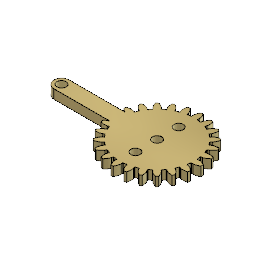
Engrenagem_v8 (Autodesk Fusion 360 design; units mm, degrees)
description: Spur Gear; Module: 1.125; Num Teeth: 24; Pressure Angle: 20.0; Backlash: 0.00 mm
Autodesk Fusion 360 part; units mm, degrees
(part 1 of 5)
sketch "Sketch1" plane through (0, 0, 0) normal (0, 1, 0) x (1, 0, 0)
sketch "Sketch1 (2)" plane through (0, 0, 0) normal (0, 0, 1) x (1, 0, 0) in component "Spur Gear (24 teeth)"
  circle A0 centre (0, 0) radius 12.0992
  circle A1 centre (0, 0) radius 1.5
extrude "Extrude1" add sketch "Sketch1 (2)" along normal blind 3 in component "Spur Gear (24 teeth)"
sketch "Sketch2" plane through (0, 0, 0) normal (0, 0, 1) x (1, 0, 0) in component "Spur Gear (24 teeth)"
  spline S0 degree 5 poles (12.6449, -1.0183) (12.6506, -1.0187) (12.6618, -1.0195) (12.6788, -1.0202) (12.7014, -1.0203) (12.7297, -1.0195) (12.758, -1.0178) (12.7864, -1.0156) (12.8147, -1.0131) (12.8431, -1.0105) (12.8715, -1.0076) (12.8999, -1.0045) (12.9284, -1.0011) (12.9568, -0.9973) (12.9852, -0.9932) (13.0137, -0.9886) (13.0421, -0.9838) (13.0705, -0.9787) (13.099, -0.9733) (13.1274, -0.9678) (13.1559, -0.962) (13.1843, -0.956) (13.2127, -0.9498) (13.2412, -0.9433) (13.2696, -0.9366) (13.298, -0.9297) (13.3264, -0.9226) (13.3549, -0.9152) (13.3833, -0.9076) (13.4117, -0.8999) (13.4401, -0.8919) (13.4684, -0.8838) (13.4968, -0.8754) (13.5252, -0.8669) (13.5535, -0.8581) (13.5819, -0.8492) (13.6102, -0.8401) (13.6385, -0.8308) (13.6669, -0.8214) (13.6952, -0.8117) (13.7234, -0.8019) (13.7517, -0.7919) (13.78, -0.7817) (13.8082, -0.7714) (13.8365, -0.7609) (13.8647, -0.7502) (13.8929, -0.7393) (13.9211, -0.7283) (13.9492, -0.7171) (13.9774, -0.7058) (14.0055, -0.6943) (14.0337, -0.6826) (14.0618, -0.6708) (14.0898, -0.6588) (14.1179, -0.6467) (14.146, -0.6344) (14.174, -0.6219) (14.202, -0.6093) (14.23, -0.5966) (14.2579, -0.5837) (14.2859, -0.5706) (14.3138, -0.5574) (14.3417, -0.544) (14.3696, -0.5305) (14.3975, -0.5169) (14.4253, -0.5031) (14.4531, -0.4891) (14.4809, -0.4751) (14.5087, -0.4608) (14.5364, -0.4465) (14.5641, -0.4319) (14.5863, -0.4202) (14.6029, -0.4114) (14.6139, -0.4054) (14.6195, -0.4024) knots 0 0 0 0 0 0 0.01428571 0.02857143 0.04285714 0.05714286 0.07142857 0.08571429 0.1 0.11428571 0.12857143 0.14285714 0.15714286 0.17142857 0.18571429 0.2 0.21428571 0.22857143 0.24285714 0.25714286 0.27142857 0.28571429 0.3 0.31428571 0.32857143 0.34285714 0.35714286 0.37142857 0.38571429 0.4 0.41428571 0.42857143 0.44285714 0.45714286 0.47142857 0.48571429 0.5 0.51428571 0.52857143 0.54285714 0.55714286 0.57142857 0.58571429 0.6 0.61428571 0.62857143 0.64285714 0.65714286 0.67142857 0.68571429 0.7 0.71428571 0.72857143 0.74285714 0.75714286 0.77142857 0.78571429 0.8 0.81428571 0.82857143 0.84285714 0.85714286 0.87142857 0.88571429 0.9 0.91428571 0.92857143 0.94285714 0.95714286 0.97142857 0.98571429 1 1 1 1 1 1
  spline S1 degree 5 poles (12.6449, 1.0183) (12.6506, 1.0187) (12.6618, 1.0195) (12.6788, 1.0202) (12.7014, 1.0203) (12.7297, 1.0195) (12.758, 1.0178) (12.7864, 1.0156) (12.8147, 1.0131) (12.8431, 1.0105) (12.8715, 1.0076) (12.8999, 1.0045) (12.9284, 1.0011) (12.9568, 0.9973) (12.9852, 0.9932) (13.0137, 0.9886) (13.0421, 0.9838) (13.0705, 0.9787) (13.099, 0.9733) (13.1274, 0.9678) (13.1559, 0.962) (13.1843, 0.956) (13.2127, 0.9498) (13.2412, 0.9433) (13.2696, 0.9366) (13.298, 0.9297) (13.3264, 0.9226) (13.3549, 0.9152) (13.3833, 0.9076) (13.4117, 0.8999) (13.4401, 0.8919) (13.4684, 0.8838) (13.4968, 0.8754) (13.5252, 0.8669) (13.5535, 0.8581) (13.5819, 0.8492) (13.6102, 0.8401) (13.6385, 0.8308) (13.6669, 0.8214) (13.6952, 0.8117) (13.7234, 0.8019) (13.7517, 0.7919) (13.78, 0.7817) (13.8082, 0.7714) (13.8365, 0.7609) (13.8647, 0.7502) (13.8929, 0.7393) (13.9211, 0.7283) (13.9492, 0.7171) (13.9774, 0.7058) (14.0055, 0.6943) (14.0337, 0.6826) (14.0618, 0.6708) (14.0898, 0.6588) (14.1179, 0.6467) (14.146, 0.6344) (14.174, 0.6219) (14.202, 0.6093) (14.23, 0.5966) (14.2579, 0.5837) (14.2859, 0.5706) (14.3138, 0.5574) (14.3417, 0.544) (14.3696, 0.5305) (14.3975, 0.5169) (14.4253, 0.5031) (14.4531, 0.4891) (14.4809, 0.4751) (14.5087, 0.4608) (14.5364, 0.4465) (14.5641, 0.4319) (14.5863, 0.4202) (14.6029, 0.4114) (14.6139, 0.4054) (14.6195, 0.4024) knots 0 0 0 0 0 0 0.01428571 0.02857143 0.04285714 0.05714286 0.07142857 0.08571429 0.1 0.11428571 0.12857143 0.14285714 0.15714286 0.17142857 0.18571429 0.2 0.21428571 0.22857143 0.24285714 0.25714286 0.27142857 0.28571429 0.3 0.31428571 0.32857143 0.34285714 0.35714286 0.37142857 0.38571429 0.4 0.41428571 0.42857143 0.44285714 0.45714286 0.47142857 0.48571429 0.5 0.51428571 0.52857143 0.54285714 0.55714286 0.57142857 0.58571429 0.6 0.61428571 0.62857143 0.64285714 0.65714286 0.67142857 0.68571429 0.7 0.71428571 0.72857143 0.74285714 0.75714286 0.77142857 0.78571429 0.8 0.81428571 0.82857143 0.84285714 0.85714286 0.87142857 0.88571429 0.9 0.91428571 0.92857143 0.94285714 0.95714286 0.97142857 0.98571429 1 1 1 1 1 1
  arc A0 (14.6195, -0.4024) -> (14.6195, 0.4024) centre (0, 0) ccw
  line L0 (12.0502, -0.9712) -> (12.6449, -1.0183)
  line L1 (12.0502, 0.9712) -> (12.6449, 1.0183)
  line L2 (12.0502, -0.9712) -> (12.0502, 0.9712)
  point P0 (12.7841, -1.0157)
  point P1 (12.9241, -1.0016)
  point P2 (13.0647, -0.9797)
  point P3 (13.2057, -0.9513)
  point P4 (13.3469, -0.9172)
  point P5 (13.4884, -0.8779)
  point P6 (13.63, -0.8336)
  point P7 (13.7716, -0.7847)
  point P8 (13.9132, -0.7313)
  point P9 (14.0548, -0.6737)
  point P10 (14.1963, -0.6119)
  point P11 (14.3376, -0.546)
  point P12 (14.4787, -0.4761)
  point P13 (12.7841, 1.0157)
  point P14 (12.9241, 1.0016)
  point P15 (13.0647, 0.9797)
  point P16 (13.2057, 0.9513)
  point P17 (13.3469, 0.9172)
  point P18 (13.4884, 0.8779)
  point P19 (13.63, 0.8336)
  point P20 (13.7716, 0.7847)
  point P21 (13.9132, 0.7313)
  point P22 (14.0548, 0.6737)
  point P23 (14.1963, 0.6119)
  point P24 (14.3376, 0.546)
  point P25 (14.4787, 0.4761)
extrude "Extrude2" add sketch "Sketch2" along normal blind 3 in component "Spur Gear (24 teeth)"
fillet "Fillet1" radius 0.1 2 edges at (12.0601, -0.972, 1.5) (12.0601, 0.972, 1.5) in component "Spur Gear (24 teeth)"
pattern_circular "C-Pattern1" count 24 over 360 about axis through (0, 0, 0) along (0, 0, 1) of "Extrude2", "Fillet1" in component "Spur Gear (24 teeth)"
sketch "Sketch3" plane through (0, 0, 0) normal (0, 0, 1) x (1, 0, 0) in component "Spur Gear (24 teeth)"
  circle A0 centre (0, 0) radius 13.5 construction
sketch "Sketch2 (2)" plane through (0, 0, 3) normal (0, 0, 1) x (1, 0, 0)
  arc A0 (11.9182, -2.0851) -> (12.0517, -1.0706) centre (0, 0) ccw
  arc A1 (12.1592, -0.9798) -> (12.0517, -1.0706) centre (12.1513, -1.0795) ccw
  line L0 (12.1592, -0.9798) -> (12.6449, -1.0183)
  spline S0 degree 5 poles (12.6449, -1.0183) (12.6506, -1.0187) (12.6618, -1.0195) (12.6788, -1.0202) (12.7014, -1.0203) (12.7297, -1.0195) (12.758, -1.0178) (12.7864, -1.0156) (12.8147, -1.0131) (12.8431, -1.0105) (12.8715, -1.0076) (12.8999, -1.0045) (12.9284, -1.0011) (12.9568, -0.9973) (12.9852, -0.9932) (13.0137, -0.9886) (13.0421, -0.9838) (13.0705, -0.9787) (13.099, -0.9733) (13.1274, -0.9678) (13.1559, -0.962) (13.1843, -0.956) (13.2127, -0.9498) (13.2412, -0.9433) (13.2696, -0.9366) (13.298, -0.9297) (13.3264, -0.9226) (13.3549, -0.9152) (13.3833, -0.9076) (13.4117, -0.8999) (13.4401, -0.8919) (13.4684, -0.8838) (13.4968, -0.8754) (13.5252, -0.8669) (13.5535, -0.8581) (13.5819, -0.8492) (13.6102, -0.8401) (13.6385, -0.8308) (13.6669, -0.8214) (13.6952, -0.8117) (13.7234, -0.8019) (13.7517, -0.7919) (13.78, -0.7817) (13.8082, -0.7714) (13.8365, -0.7609) (13.8647, -0.7502) (13.8929, -0.7393) (13.9211, -0.7283) (13.9492, -0.7171) (13.9774, -0.7058) (14.0055, -0.6943) (14.0337, -0.6826) (14.0618, -0.6708) (14.0898, -0.6588) (14.1179, -0.6467) (14.146, -0.6344) (14.174, -0.6219) (14.202, -0.6093) (14.23, -0.5966) (14.2579, -0.5837) (14.2859, -0.5706) (14.3138, -0.5574) (14.3417, -0.544) (14.3696, -0.5305) (14.3975, -0.5169) (14.4253, -0.5031) (14.4531, -0.4891) (14.4809, -0.4751) (14.5087, -0.4608) (14.5364, -0.4465) (14.5641, -0.4319) (14.5863, -0.4202) (14.6029, -0.4114) (14.6139, -0.4054) (14.6195, -0.4024) knots 0 0 0 0 0 0 0.01428571 0.02857143 0.04285714 0.05714286 0.07142857 0.08571429 0.1 0.11428571 0.12857143 0.14285714 0.15714286 0.17142857 0.18571429 0.2 0.21428571 0.22857143 0.24285714 0.25714286 0.27142857 0.28571429 0.3 0.31428571 0.32857143 0.34285714 0.35714286 0.37142857 0.38571429 0.4 0.41428571 0.42857143 0.44285714 0.45714286 0.47142857 0.48571429 0.5 0.51428571 0.52857143 0.54285714 0.55714286 0.57142857 0.58571429 0.6 0.61428571 0.62857143 0.64285714 0.65714286 0.67142857 0.68571429 0.7 0.71428571 0.72857143 0.74285714 0.75714286 0.77142857 0.78571429 0.8 0.81428571 0.82857143 0.84285714 0.85714286 0.87142857 0.88571429 0.9 0.91428571 0.92857143 0.94285714 0.95714286 0.97142857 0.98571429 1 1 1 1 1 1
  arc A2 (14.6195, -0.4024) -> (14.6195, 0.4024) centre (0, 0) ccw
  spline S1 degree 5 poles (14.6195, 0.4024) (14.6139, 0.4054) (14.6029, 0.4114) (14.5863, 0.4202) (14.5641, 0.4319) (14.5364, 0.4465) (14.5087, 0.4608) (14.4809, 0.4751) (14.4531, 0.4891) (14.4253, 0.5031) (14.3975, 0.5169) (14.3696, 0.5305) (14.3417, 0.544) (14.3138, 0.5574) (14.2859, 0.5706) (14.2579, 0.5837) (14.23, 0.5966) (14.202, 0.6093) (14.174, 0.6219) (14.146, 0.6344) (14.1179, 0.6467) (14.0898, 0.6588) (14.0618, 0.6708) (14.0337, 0.6826) (14.0055, 0.6943) (13.9774, 0.7058) (13.9492, 0.7171) (13.9211, 0.7283) (13.8929, 0.7393) (13.8647, 0.7502) (13.8365, 0.7609) (13.8082, 0.7714) (13.78, 0.7817) (13.7517, 0.7919) (13.7234, 0.8019) (13.6952, 0.8117) (13.6669, 0.8214) (13.6385, 0.8308) (13.6102, 0.8401) (13.5819, 0.8492) (13.5535, 0.8581) (13.5252, 0.8669) (13.4968, 0.8754) (13.4684, 0.8838) (13.4401, 0.8919) (13.4117, 0.8999) (13.3833, 0.9076) (13.3549, 0.9152) (13.3264, 0.9226) (13.298, 0.9297) (13.2696, 0.9366) (13.2412, 0.9433) (13.2127, 0.9498) (13.1843, 0.956) (13.1559, 0.962) (13.1274, 0.9678) (13.099, 0.9733) (13.0705, 0.9787) (13.0421, 0.9838) (13.0137, 0.9886) (12.9852, 0.9932) (12.9568, 0.9973) (12.9284, 1.0011) (12.8999, 1.0045) (12.8715, 1.0076) (12.8431, 1.0105) (12.8147, 1.0131) (12.7864, 1.0156) (12.758, 1.0178) (12.7297, 1.0195) (12.7014, 1.0203) (12.6788, 1.0202) (12.6618, 1.0195) (12.6506, 1.0187) (12.6449, 1.0183) knots -1 -1 -1 -1 -1 -1 -0.98571429 -0.97142857 -0.95714286 -0.94285714 -0.92857143 -0.91428571 -0.9 -0.88571429 -0.87142857 -0.85714286 -0.84285714 -0.82857143 -0.81428571 -0.8 -0.78571429 -0.77142857 -0.75714286 -0.74285714 -0.72857143 -0.71428571 -0.7 -0.68571429 -0.67142857 -0.65714286 -0.64285714 -0.62857143 -0.61428571 -0.6 -0.58571429 -0.57142857 -0.55714286 -0.54285714 -0.52857143 -0.51428571 -0.5 -0.48571429 -0.47142857 -0.45714286 -0.44285714 -0.42857143 -0.41428571 -0.4 -0.38571429 -0.37142857 -0.35714286 -0.34285714 -0.32857143 -0.31428571 -0.3 -0.28571429 -0.27142857 -0.25714286 -0.24285714 -0.22857143 -0.21428571 -0.2 -0.18571429 -0.17142857 -0.15714286 -0.14285714 -0.12857143 -0.11428571 -0.1 -0.08571429 -0.07142857 -0.05714286 -0.04285714 -0.02857143 -0.01428571 0 0 0 0 0 0
  line L1 (12.6449, 1.0183) -> (12.1592, 0.9798)
  arc A3 (12.0517, 1.0706) -> (12.1592, 0.9798) centre (12.1513, 1.0795) ccw
  arc A4 (12.0517, 1.0706) -> (11.9182, 2.0851) centre (0, 0) ccw
  arc A5 (11.9985, 2.2006) -> (11.9182, 2.0851) centre (12.0167, 2.1023) ccw
  line L2 (11.9985, 2.2006) -> (12.4776, 2.2892)
  spline S2 degree 5 poles (12.4776, 2.2892) (12.4832, 2.2902) (12.4943, 2.2924) (12.5108, 2.2961) (12.5327, 2.3018) (12.5598, 2.31) (12.5867, 2.3189) (12.6135, 2.3284) (12.6403, 2.3381) (12.667, 2.348) (12.6937, 2.3581) (12.7204, 2.3684) (12.747, 2.3791) (12.7734, 2.3901) (12.7998, 2.4015) (12.8261, 2.4133) (12.8523, 2.4253) (12.8785, 2.4376) (12.9046, 2.4501) (12.9306, 2.4628) (12.9566, 2.4758) (12.9825, 2.4889) (13.0083, 2.5023) (13.0341, 2.5159) (13.0599, 2.5297) (13.0855, 2.5438) (13.1111, 2.558) (13.1367, 2.5725) (13.1621, 2.5871) (13.1876, 2.602) (13.2129, 2.617) (13.2382, 2.6322) (13.2635, 2.6476) (13.2887, 2.6632) (13.3138, 2.679) (13.3389, 2.695) (13.3639, 2.7111) (13.3889, 2.7274) (13.4138, 2.7439) (13.4386, 2.7605) (13.4634, 2.7773) (13.4881, 2.7943) (13.5128, 2.8114) (13.5374, 2.8287) (13.5619, 2.8462) (13.5864, 2.8638) (13.6108, 2.8816) (13.6352, 2.8996) (13.6595, 2.9176) (13.6838, 2.9359) (13.708, 2.9543) (13.7321, 2.9728) (13.7562, 2.9915) (13.7803, 3.0104) (13.8042, 3.0294) (13.8281, 3.0485) (13.852, 3.0678) (13.8758, 3.0872) (13.8995, 3.1068) (13.9232, 3.1265) (13.9468, 3.1463) (13.9703, 3.1663) (13.9938, 3.1864) (14.0173, 3.2067) (14.0406, 3.2271) (14.064, 3.2476) (14.0872, 3.2683) (14.1104, 3.2891) (14.1336, 3.31) (14.1566, 3.3311) (14.1796, 3.3522) (14.198, 3.3693) (14.2118, 3.3822) (14.2209, 3.3908) (14.2255, 3.3951) knots 0 0 0 0 0 0 0.01428571 0.02857143 0.04285714 0.05714286 0.07142857 0.08571429 0.1 0.11428571 0.12857143 0.14285714 0.15714286 0.17142857 0.18571429 0.2 0.21428571 0.22857143 0.24285714 0.25714286 0.27142857 0.28571429 0.3 0.31428571 0.32857143 0.34285714 0.35714286 0.37142857 0.38571429 0.4 0.41428571 0.42857143 0.44285714 0.45714286 0.47142857 0.48571429 0.5 0.51428571 0.52857143 0.54285714 0.55714286 0.57142857 0.58571429 0.6 0.61428571 0.62857143 0.64285714 0.65714286 0.67142857 0.68571429 0.7 0.71428571 0.72857143 0.74285714 0.75714286 0.77142857 0.78571429 0.8 0.81428571 0.82857143 0.84285714 0.85714286 0.87142857 0.88571429 0.9 0.91428571 0.92857143 0.94285714 0.95714286 0.97142857 0.98571429 1 1 1 1 1 1
  arc A6 (14.2255, 3.3951) -> (14.0172, 4.1725) centre (0, 0) ccw
  spline S3 degree 5 poles (14.0172, 4.1725) (14.011, 4.174) (13.9988, 4.1768) (13.9805, 4.1811) (13.9561, 4.1867) (13.9255, 4.1935) (13.895, 4.2002) (13.8645, 4.2068) (13.834, 4.2132) (13.8036, 4.2195) (13.7731, 4.2256) (13.7427, 4.2316) (13.7122, 4.2374) (13.6818, 4.2431) (13.6514, 4.2486) (13.6211, 4.254) (13.5907, 4.2592) (13.5604, 4.2643) (13.53, 4.2692) (13.4998, 4.274) (13.4695, 4.2786) (13.4392, 4.2831) (13.409, 4.2874) (13.3788, 4.2915) (13.3486, 4.2955) (13.3185, 4.2993) (13.2883, 4.303) (13.2582, 4.3065) (13.2281, 4.3099) (13.1981, 4.3131) (13.1681, 4.3161) (13.1381, 4.3189) (13.1081, 4.3216) (13.0782, 4.3241) (13.0483, 4.3264) (13.0184, 4.3286) (12.9886, 4.3306) (12.9588, 4.3324) (12.929, 4.3341) (12.8993, 4.3355) (12.8696, 4.3368) (12.84, 4.3379) (12.8103, 4.3388) (12.7808, 4.3395) (12.7512, 4.3401) (12.7218, 4.3404) (12.6923, 4.3405) (12.6629, 4.3405) (12.6336, 4.3403) (12.6043, 4.3398) (12.575, 4.3391) (12.5458, 4.3383) (12.5167, 4.3371) (12.4876, 4.3358) (12.4586, 4.3342) (12.4296, 4.3324) (12.4007, 4.3304) (12.3719, 4.3282) (12.3431, 4.3258) (12.3144, 4.3231) (12.2857, 4.3201) (12.2572, 4.3168) (12.2287, 4.3131) (12.2004, 4.3091) (12.1722, 4.3047) (12.144, 4.3001) (12.1159, 4.2953) (12.0878, 4.2903) (12.0599, 4.2851) (12.0321, 4.2794) (12.0045, 4.2729) (11.9827, 4.2669) (11.9665, 4.2619) (11.9558, 4.2582) (11.9505, 4.2563) knots -1 -1 -1 -1 -1 -1 -0.98571429 -0.97142857 -0.95714286 -0.94285714 -0.92857143 -0.91428571 -0.9 -0.88571429 -0.87142857 -0.85714286 -0.84285714 -0.82857143 -0.81428571 -0.8 -0.78571429 -0.77142857 -0.75714286 -0.74285714 -0.72857143 -0.71428571 -0.7 -0.68571429 -0.67142857 -0.65714286 -0.64285714 -0.62857143 -0.61428571 -0.6 -0.58571429 -0.57142857 -0.55714286 -0.54285714 -0.52857143 -0.51428571 -0.5 -0.48571429 -0.47142857 -0.45714286 -0.44285714 -0.42857143 -0.41428571 -0.4 -0.38571429 -0.37142857 -0.35714286 -0.34285714 -0.32857143 -0.31428571 -0.3 -0.28571429 -0.27142857 -0.25714286 -0.24285714 -0.22857143 -0.21428571 -0.2 -0.18571429 -0.17142857 -0.15714286 -0.14285714 -0.12857143 -0.11428571 -0.1 -0.08571429 -0.07142857 -0.05714286 -0.04285714 -0.02857143 -0.01428571 0 0 0 0 0 0
  line L3 (11.9505, 4.2563) -> (11.4913, 4.0935)
  arc A7 (11.364, 4.1534) -> (11.4913, 4.0935) centre (11.4579, 4.1877) ccw
  arc A8 (11.364, 4.1534) -> (10.9724, 5.0987) centre (0, 0) ccw
  arc A9 (11.0201, 5.2311) -> (10.9724, 5.0987) centre (11.0631, 5.1408) ccw
  line L4 (11.0201, 5.2311) -> (11.46, 5.4406)
  spline S4 degree 5 poles (11.46, 5.4406) (11.4651, 5.443) (11.4752, 5.448) (11.4902, 5.4559) (11.5099, 5.4671) (11.534, 5.482) (11.5577, 5.4976) (11.5811, 5.5137) (11.6045, 5.53) (11.6277, 5.5465) (11.6509, 5.5631) (11.674, 5.58) (11.6969, 5.5972) (11.7196, 5.6147) (11.7421, 5.6325) (11.7645, 5.6507) (11.7867, 5.6691) (11.8087, 5.6877) (11.8307, 5.7066) (11.8526, 5.7256) (11.8743, 5.7448) (11.8959, 5.7642) (11.9175, 5.7838) (11.9389, 5.8036) (11.9601, 5.8236) (11.9813, 5.8439) (12.0023, 5.8643) (12.0232, 5.8848) (12.0441, 5.9056) (12.0648, 5.9265) (12.0854, 5.9476) (12.1059, 5.9689) (12.1263, 5.9903) (12.1466, 6.0119) (12.1668, 6.0336) (12.1869, 6.0555) (12.2069, 6.0775) (12.2267, 6.0998) (12.2465, 6.1221) (12.2662, 6.1446) (12.2858, 6.1673) (12.3053, 6.1901) (12.3247, 6.213) (12.344, 6.2361) (12.3632, 6.2593) (12.3822, 6.2827) (12.4012, 6.3062) (12.4202, 6.3298) (12.439, 6.3536) (12.4577, 6.3775) (12.4763, 6.4015) (12.4948, 6.4257) (12.5132, 6.45) (12.5316, 6.4744) (12.5498, 6.4989) (12.5679, 6.5236) (12.586, 6.5484) (12.6039, 6.5733) (12.6218, 6.5983) (12.6396, 6.6235) (12.6572, 6.6488) (12.6748, 6.6742) (12.6923, 6.6997) (12.7097, 6.7253) (12.727, 6.7511) (12.7442, 6.777) (12.7613, 6.8029) (12.7783, 6.829) (12.7953, 6.8552) (12.8121, 6.8816) (12.8289, 6.908) (12.8422, 6.9292) (12.8521, 6.9452) (12.8587, 6.9559) (12.862, 6.9612) knots 0 0 0 0 0 0 0.01428571 0.02857143 0.04285714 0.05714286 0.07142857 0.08571429 0.1 0.11428571 0.12857143 0.14285714 0.15714286 0.17142857 0.18571429 0.2 0.21428571 0.22857143 0.24285714 0.25714286 0.27142857 0.28571429 0.3 0.31428571 0.32857143 0.34285714 0.35714286 0.37142857 0.38571429 0.4 0.41428571 0.42857143 0.44285714 0.45714286 0.47142857 0.48571429 0.5 0.51428571 0.52857143 0.54285714 0.55714286 0.57142857 0.58571429 0.6 0.61428571 0.62857143 0.64285714 0.65714286 0.67142857 0.68571429 0.7 0.71428571 0.72857143 0.74285714 0.75714286 0.77142857 0.78571429 0.8 0.81428571 0.82857143 0.84285714 0.85714286 0.87142857 0.88571429 0.9 0.91428571 0.92857143 0.94285714 0.95714286 0.97142857 0.98571429 1 1 1 1 1 1
  arc A10 (12.862, 6.9612) -> (12.4596, 7.6583) centre (0, 0) ccw
  spline S5 degree 5 poles (12.4596, 7.6583) (12.4533, 7.6581) (12.4408, 7.6577) (12.422, 7.657) (12.3969, 7.6561) (12.3657, 7.6548) (12.3344, 7.6534) (12.3033, 7.6519) (12.2722, 7.6502) (12.2411, 7.6483) (12.2101, 7.6464) (12.1792, 7.6442) (12.1483, 7.642) (12.1174, 7.6396) (12.0866, 7.6371) (12.0559, 7.6344) (12.0252, 7.6316) (11.9946, 7.6287) (11.9641, 7.6256) (11.9336, 7.6224) (11.9031, 7.619) (11.8728, 7.6155) (11.8424, 7.6118) (11.8122, 7.608) (11.782, 7.604) (11.7519, 7.5999) (11.7218, 7.5957) (11.6918, 7.5913) (11.6619, 7.5867) (11.6321, 7.582) (11.6023, 7.5771) (11.5726, 7.5721) (11.543, 7.567) (11.5134, 7.5617) (11.4839, 7.5562) (11.4545, 7.5505) (11.4252, 7.5447) (11.3959, 7.5388) (11.3667, 7.5327) (11.3376, 7.5264) (11.3086, 7.5199) (11.2797, 7.5133) (11.2509, 7.5065) (11.2221, 7.4996) (11.1935, 7.4924) (11.1649, 7.4851) (11.1364, 7.4777) (11.108, 7.47) (11.0798, 7.4622) (11.0516, 7.4542) (11.0235, 7.4459) (10.9955, 7.4375) (10.9677, 7.4289) (10.9399, 7.4201) (10.9123, 7.411) (10.8848, 7.4018) (10.8574, 7.3924) (10.8301, 7.3828) (10.8029, 7.373) (10.7759, 7.363) (10.749, 7.3527) (10.7222, 7.3421) (10.6957, 7.3312) (10.6694, 7.3199) (10.6433, 7.3084) (10.6172, 7.2967) (10.5913, 7.2848) (10.5655, 7.2727) (10.5399, 7.2604) (10.5145, 7.2477) (10.4896, 7.2343) (10.4701, 7.2229) (10.4557, 7.2138) (10.4463, 7.2075) (10.4417, 7.2043) knots -1 -1 -1 -1 -1 -1 -0.98571429 -0.97142857 -0.95714286 -0.94285714 -0.92857143 -0.91428571 -0.9 -0.88571429 -0.87142857 -0.85714286 -0.84285714 -0.82857143 -0.81428571 -0.8 -0.78571429 -0.77142857 -0.75714286 -0.74285714 -0.72857143 -0.71428571 -0.7 -0.68571429 -0.67142857 -0.65714286 -0.64285714 -0.62857143 -0.61428571 -0.6 -0.58571429 -0.57142857 -0.55714286 -0.54285714 -0.52857143 -0.51428571 -0.5 -0.48571429 -0.47142857 -0.45714286 -0.44285714 -0.42857143 -0.41428571 -0.4 -0.38571429 -0.37142857 -0.35714286 -0.34285714 -0.32857143 -0.31428571 -0.3 -0.28571429 -0.27142857 -0.25714286 -0.24285714 -0.22857143 -0.21428571 -0.2 -0.18571429 -0.17142857 -0.15714286 -0.14285714 -0.12857143 -0.11428571 -0.1 -0.08571429 -0.07142857 -0.05714286 -0.04285714 -0.02857143 -0.01428571 0 0 0 0 0 0
  line L5 (10.4417, 7.2043) -> (10.0403, 6.9282)
  arc A11 (9.9018, 6.9531) -> (10.0403, 6.9282) centre (9.9836, 7.0105) ccw
  arc A12 (9.9018, 6.9531) -> (9.2789, 7.7648) centre (0, 0) ccw
  arc A13 (9.2907, 7.905) -> (9.2789, 7.7648) centre (9.3556, 7.829) ccw
  line L6 (9.2907, 7.905) -> (9.6613, 8.2213)
  spline S6 degree 5 poles (9.6613, 8.2213) (9.6656, 8.225) (9.6741, 8.2324) (9.6866, 8.2439) (9.7027, 8.2597) (9.7221, 8.2804) (9.741, 8.3016) (9.7595, 8.3232) (9.7778, 8.345) (9.796, 8.367) (9.8141, 8.3891) (9.832, 8.4113) (9.8496, 8.4338) (9.8671, 8.4566) (9.8842, 8.4797) (9.9011, 8.503) (9.9178, 8.5265) (9.9343, 8.5503) (9.9506, 8.5741) (9.9668, 8.5982) (9.9828, 8.6224) (9.9987, 8.6467) (10.0144, 8.6712) (10.03, 8.6959) (10.0453, 8.7207) (10.0605, 8.7457) (10.0756, 8.7709) (10.0904, 8.7962) (10.1052, 8.8216) (10.1198, 8.8472) (10.1342, 8.8729) (10.1485, 8.8987) (10.1627, 8.9247) (10.1767, 8.9508) (10.1906, 8.977) (10.2043, 9.0033) (10.2179, 9.0298) (10.2314, 9.0564) (10.2447, 9.0831) (10.2579, 9.11) (10.271, 9.1369) (10.2839, 9.164) (10.2967, 9.1912) (10.3093, 9.2185) (10.3219, 9.2459) (10.3343, 9.2734) (10.3465, 9.301) (10.3587, 9.3287) (10.3707, 9.3565) (10.3826, 9.3845) (10.3943, 9.4125) (10.406, 9.4406) (10.4175, 9.4688) (10.4289, 9.4972) (10.4401, 9.5256) (10.4513, 9.5541) (10.4623, 9.5828) (10.4732, 9.6115) (10.4839, 9.6403) (10.4946, 9.6692) (10.5051, 9.6982) (10.5155, 9.7273) (10.5258, 9.7564) (10.536, 9.7857) (10.546, 9.815) (10.556, 9.8445) (10.5658, 9.874) (10.5754, 9.9036) (10.585, 9.9333) (10.5945, 9.9631) (10.6038, 9.993) (10.6112, 10.0169) (10.6167, 10.0349) (10.6203, 10.0469) (10.6221, 10.0529) knots 0 0 0 0 0 0 0.01428571 0.02857143 0.04285714 0.05714286 0.07142857 0.08571429 0.1 0.11428571 0.12857143 0.14285714 0.15714286 0.17142857 0.18571429 0.2 0.21428571 0.22857143 0.24285714 0.25714286 0.27142857 0.28571429 0.3 0.31428571 0.32857143 0.34285714 0.35714286 0.37142857 0.38571429 0.4 0.41428571 0.42857143 0.44285714 0.45714286 0.47142857 0.48571429 0.5 0.51428571 0.52857143 0.54285714 0.55714286 0.57142857 0.58571429 0.6 0.61428571 0.62857143 0.64285714 0.65714286 0.67142857 0.68571429 0.7 0.71428571 0.72857143 0.74285714 0.75714286 0.77142857 0.78571429 0.8 0.81428571 0.82857143 0.84285714 0.85714286 0.87142857 0.88571429 0.9 0.91428571 0.92857143 0.94285714 0.95714286 0.97142857 0.98571429 1 1 1 1 1 1
  arc A14 (10.6221, 10.0529) -> (10.0529, 10.6221) centre (0, 0) ccw
  spline S7 degree 5 poles (10.0529, 10.6221) (10.0469, 10.6203) (10.0349, 10.6167) (10.0169, 10.6112) (9.993, 10.6038) (9.9631, 10.5945) (9.9333, 10.585) (9.9036, 10.5754) (9.874, 10.5658) (9.8445, 10.556) (9.815, 10.546) (9.7857, 10.536) (9.7564, 10.5258) (9.7273, 10.5155) (9.6982, 10.5051) (9.6692, 10.4946) (9.6403, 10.4839) (9.6115, 10.4732) (9.5828, 10.4623) (9.5541, 10.4513) (9.5256, 10.4401) (9.4972, 10.4289) (9.4688, 10.4175) (9.4406, 10.406) (9.4125, 10.3943) (9.3845, 10.3826) (9.3565, 10.3707) (9.3287, 10.3587) (9.301, 10.3465) (9.2734, 10.3343) (9.2459, 10.3219) (9.2185, 10.3093) (9.1912, 10.2967) (9.164, 10.2839) (9.1369, 10.271) (9.11, 10.2579) (9.0831, 10.2447) (9.0564, 10.2314) (9.0298, 10.2179) (9.0033, 10.2043) (8.977, 10.1906) (8.9508, 10.1767) (8.9247, 10.1627) (8.8987, 10.1485) (8.8729, 10.1342) (8.8472, 10.1198) (8.8216, 10.1052) (8.7962, 10.0904) (8.7709, 10.0756) (8.7457, 10.0605) (8.7207, 10.0453) (8.6959, 10.03) (8.6712, 10.0144) (8.6467, 9.9987) (8.6224, 9.9828) (8.5982, 9.9668) (8.5741, 9.9506) (8.5503, 9.9343) (8.5265, 9.9178) (8.503, 9.9011) (8.4797, 9.8842) (8.4566, 9.8671) (8.4338, 9.8496) (8.4113, 9.832) (8.3891, 9.8141) (8.367, 9.796) (8.345, 9.7778) (8.3232, 9.7595) (8.3016, 9.741) (8.2804, 9.7221) (8.2597, 9.7027) (8.2439, 9.6866) (8.2324, 9.6741) (8.225, 9.6656) (8.2213, 9.6613) knots -1 -1 -1 -1 -1 -1 -0.98571429 -0.97142857 -0.95714286 -0.94285714 -0.92857143 -0.91428571 -0.9 -0.88571429 -0.87142857 -0.85714286 -0.84285714 -0.82857143 -0.81428571 -0.8 -0.78571429 -0.77142857 -0.75714286 -0.74285714 -0.72857143 -0.71428571 -0.7 -0.68571429 -0.67142857 -0.65714286 -0.64285714 -0.62857143 -0.61428571 -0.6 -0.58571429 -0.57142857 -0.55714286 -0.54285714 -0.52857143 -0.51428571 -0.5 -0.48571429 -0.47142857 -0.45714286 -0.44285714 -0.42857143 -0.41428571 -0.4 -0.38571429 -0.37142857 -0.35714286 -0.34285714 -0.32857143 -0.31428571 -0.3 -0.28571429 -0.27142857 -0.25714286 -0.24285714 -0.22857143 -0.21428571 -0.2 -0.18571429 -0.17142857 -0.15714286 -0.14285714 -0.12857143 -0.11428571 -0.1 -0.08571429 -0.07142857 -0.05714286 -0.04285714 -0.02857143 -0.01428571 0 0 0 0 0 0
  line L7 (8.2213, 9.6613) -> (7.905, 9.2907)
  arc A15 (7.7648, 9.2789) -> (7.905, 9.2907) centre (7.829, 9.3556) ccw
  arc A16 (7.7648, 9.2789) -> (6.9531, 9.9018) centre (0, 0) ccw
  arc A17 (6.9282, 10.0403) -> (6.9531, 9.9018) centre (7.0105, 9.9836) ccw
  line L8 (6.9282, 10.0403) -> (7.2043, 10.4417)
  spline S8 degree 5 poles (7.2043, 10.4417) (7.2075, 10.4463) (7.2138, 10.4557) (7.2229, 10.4701) (7.2343, 10.4896) (7.2477, 10.5145) (7.2604, 10.5399) (7.2727, 10.5655) (7.2848, 10.5913) (7.2967, 10.6172) (7.3084, 10.6433) (7.3199, 10.6694) (7.3312, 10.6957) (7.3421, 10.7222) (7.3527, 10.749) (7.363, 10.7759) (7.373, 10.8029) (7.3828, 10.8301) (7.3924, 10.8574) (7.4018, 10.8848) (7.411, 10.9123) (7.4201, 10.9399) (7.4289, 10.9677) (7.4375, 10.9955) (7.4459, 11.0235) (7.4542, 11.0516) (7.4622, 11.0798) (7.47, 11.108) (7.4777, 11.1364) (7.4851, 11.1649) (7.4924, 11.1935) (7.4996, 11.2221) (7.5065, 11.2509) (7.5133, 11.2797) (7.5199, 11.3086) (7.5264, 11.3376) (7.5327, 11.3667) (7.5388, 11.3959) (7.5447, 11.4252) (7.5505, 11.4545) (7.5562, 11.4839) (7.5617, 11.5134) (7.567, 11.543) (7.5721, 11.5726) (7.5771, 11.6023) (7.582, 11.6321) (7.5867, 11.6619) (7.5913, 11.6918) (7.5957, 11.7218) (7.5999, 11.7519) (7.604, 11.782) (7.608, 11.8122) (7.6118, 11.8424) (7.6155, 11.8728) (7.619, 11.9031) (7.6224, 11.9336) (7.6256, 11.9641) (7.6287, 11.9946) (7.6316, 12.0252) (7.6344, 12.0559) (7.6371, 12.0866) (7.6396, 12.1174) (7.642, 12.1483) (7.6442, 12.1792) (7.6464, 12.2101) (7.6483, 12.2411) (7.6502, 12.2722) (7.6519, 12.3033) (7.6534, 12.3344) (7.6548, 12.3657) (7.6561, 12.3969) (7.657, 12.422) (7.6577, 12.4408) (7.6581, 12.4533) (7.6583, 12.4596) knots 0 0 0 0 0 0 0.01428571 0.02857143 0.04285714 0.05714286 0.07142857 0.08571429 0.1 0.11428571 0.12857143 0.14285714 0.15714286 0.17142857 0.18571429 0.2 0.21428571 0.22857143 0.24285714 0.25714286 0.27142857 0.28571429 0.3 0.31428571 0.32857143 0.34285714 0.35714286 0.37142857 0.38571429 0.4 0.41428571 0.42857143 0.44285714 0.45714286 0.47142857 0.48571429 0.5 0.51428571 0.52857143 0.54285714 0.55714286 0.57142857 0.58571429 0.6 0.61428571 0.62857143 0.64285714 0.65714286 0.67142857 0.68571429 0.7 0.71428571 0.72857143 0.74285714 0.75714286 0.77142857 0.78571429 0.8 0.81428571 0.82857143 0.84285714 0.85714286 0.87142857 0.88571429 0.9 0.91428571 0.92857143 0.94285714 0.95714286 0.97142857 0.98571429 1 1 1 1 1 1
  arc A18 (7.6583, 12.4596) -> (6.9612, 12.862) centre (0, 0) ccw
  spline S9 degree 5 poles (6.9612, 12.862) (6.9559, 12.8587) (6.9452, 12.8521) (6.9292, 12.8422) (6.908, 12.8289) (6.8816, 12.8121) (6.8552, 12.7953) (6.829, 12.7783) (6.8029, 12.7613) (6.777, 12.7442) (6.7511, 12.727) (6.7253, 12.7097) (6.6997, 12.6923) (6.6742, 12.6748) (6.6488, 12.6572) (6.6235, 12.6396) (6.5983, 12.6218) (6.5733, 12.6039) (6.5484, 12.586) (6.5236, 12.5679) (6.4989, 12.5498) (6.4744, 12.5316) (6.45, 12.5132) (6.4257, 12.4948) (6.4015, 12.4763) (6.3775, 12.4577) (6.3536, 12.439) (6.3298, 12.4202) (6.3062, 12.4012) (6.2827, 12.3822) (6.2593, 12.3632) (6.2361, 12.344) (6.213, 12.3247) (6.1901, 12.3053) (6.1673, 12.2858) (6.1446, 12.2662) (6.1221, 12.2465) (6.0998, 12.2267) (6.0775, 12.2069) (6.0555, 12.1869) (6.0336, 12.1668) (6.0119, 12.1466) (5.9903, 12.1263) (5.9689, 12.1059) (5.9476, 12.0854) (5.9265, 12.0648) (5.9056, 12.0441) (5.8848, 12.0232) (5.8643, 12.0023) (5.8439, 11.9813) (5.8236, 11.9601) (5.8036, 11.9389) (5.7838, 11.9175) (5.7642, 11.8959) (5.7448, 11.8743) (5.7256, 11.8526) (5.7066, 11.8307) (5.6877, 11.8087) (5.6691, 11.7867) (5.6507, 11.7645) (5.6325, 11.7421) (5.6147, 11.7196) (5.5972, 11.6969) (5.58, 11.674) (5.5631, 11.6509) (5.5465, 11.6277) (5.53, 11.6045) (5.5137, 11.5811) (5.4976, 11.5577) (5.482, 11.534) (5.4671, 11.5099) (5.4559, 11.4902) (5.448, 11.4752) (5.443, 11.4651) (5.4406, 11.46) knots -1 -1 -1 -1 -1 -1 -0.98571429 -0.97142857 -0.95714286 -0.94285714 -0.92857143 -0.91428571 -0.9 -0.88571429 -0.87142857 -0.85714286 -0.84285714 -0.82857143 -0.81428571 -0.8 -0.78571429 -0.77142857 -0.75714286 -0.74285714 -0.72857143 -0.71428571 -0.7 -0.68571429 -0.67142857 -0.65714286 -0.64285714 -0.62857143 -0.61428571 -0.6 -0.58571429 -0.57142857 -0.55714286 -0.54285714 -0.52857143 -0.51428571 -0.5 -0.48571429 -0.47142857 -0.45714286 -0.44285714 -0.42857143 -0.41428571 -0.4 -0.38571429 -0.37142857 -0.35714286 -0.34285714 -0.32857143 -0.31428571 -0.3 -0.28571429 -0.27142857 -0.25714286 -0.24285714 -0.22857143 -0.21428571 -0.2 -0.18571429 -0.17142857 -0.15714286 -0.14285714 -0.12857143 -0.11428571 -0.1 -0.08571429 -0.07142857 -0.05714286 -0.04285714 -0.02857143 -0.01428571 0 0 0 0 0 0
  line L9 (5.4406, 11.46) -> (5.2311, 11.0201)
  arc A19 (5.0987, 10.9724) -> (5.2311, 11.0201) centre (5.1408, 11.0631) ccw
  arc A20 (5.0987, 10.9724) -> (4.1534, 11.364) centre (0, 0) ccw
  arc A21 (4.0935, 11.4913) -> (4.1534, 11.364) centre (4.1877, 11.4579) ccw
  line L10 (4.0935, 11.4913) -> (4.2563, 11.9505)
  spline S10 degree 5 poles (4.2563, 11.9505) (4.2582, 11.9558) (4.2619, 11.9665) (4.2669, 11.9827) (4.2729, 12.0045) (4.2794, 12.0321) (4.2851, 12.0599) (4.2903, 12.0878) (4.2953, 12.1159) (4.3001, 12.144) (4.3047, 12.1722) (4.3091, 12.2004) (4.3131, 12.2287) (4.3168, 12.2572) (4.3201, 12.2857) (4.3231, 12.3144) (4.3258, 12.3431) (4.3282, 12.3719) (4.3304, 12.4007) (4.3324, 12.4296) (4.3342, 12.4586) (4.3358, 12.4876) (4.3371, 12.5167) (4.3383, 12.5458) (4.3391, 12.575) (4.3398, 12.6043) (4.3403, 12.6336) (4.3405, 12.6629) (4.3405, 12.6923) (4.3404, 12.7218) (4.3401, 12.7512) (4.3395, 12.7808) (4.3388, 12.8103) (4.3379, 12.84) (4.3368, 12.8696) (4.3355, 12.8993) (4.3341, 12.929) (4.3324, 12.9588) (4.3306, 12.9886) (4.3286, 13.0184) (4.3264, 13.0483) (4.3241, 13.0782) (4.3216, 13.1081) (4.3189, 13.1381) (4.3161, 13.1681) (4.3131, 13.1981) (4.3099, 13.2281) (4.3065, 13.2582) (4.303, 13.2883) (4.2993, 13.3185) (4.2955, 13.3486) (4.2915, 13.3788) (4.2874, 13.409) (4.2831, 13.4392) (4.2786, 13.4695) (4.274, 13.4998) (4.2692, 13.53) (4.2643, 13.5604) (4.2592, 13.5907) (4.254, 13.6211) (4.2486, 13.6514) (4.2431, 13.6818) (4.2374, 13.7122) (4.2316, 13.7427) (4.2256, 13.7731) (4.2195, 13.8036) (4.2132, 13.834) (4.2068, 13.8645) (4.2002, 13.895) (4.1935, 13.9255) (4.1867, 13.9561) (4.1811, 13.9805) (4.1768, 13.9988) (4.174, 14.011) (4.1725, 14.0172) knots 0 0 0 0 0 0 0.01428571 0.02857143 0.04285714 0.05714286 0.07142857 0.08571429 0.1 0.11428571 0.12857143 0.14285714 0.15714286 0.17142857 0.18571429 0.2 0.21428571 0.22857143 0.24285714 0.25714286 0.27142857 0.28571429 0.3 0.31428571 0.32857143 0.34285714 0.35714286 0.37142857 0.38571429 0.4 0.41428571 0.42857143 0.44285714 0.45714286 0.47142857 0.48571429 0.5 0.51428571 0.52857143 0.54285714 0.55714286 0.57142857 0.58571429 0.6 0.61428571 0.62857143 0.64285714 0.65714286 0.67142857 0.68571429 0.7 0.71428571 0.72857143 0.74285714 0.75714286 0.77142857 0.78571429 0.8 0.81428571 0.82857143 0.84285714 0.85714286 0.87142857 0.88571429 0.9 0.91428571 0.92857143 0.94285714 0.95714286 0.97142857 0.98571429 1 1 1 1 1 1
  arc A22 (4.1725, 14.0172) -> (3.3951, 14.2255) centre (0, 0) ccw
  spline S11 degree 5 poles (3.3951, 14.2255) (3.3908, 14.2209) (3.3822, 14.2118) (3.3693, 14.198) (3.3522, 14.1796) (3.3311, 14.1566) (3.31, 14.1336) (3.2891, 14.1104) (3.2683, 14.0872) (3.2476, 14.064) (3.2271, 14.0406) (3.2067, 14.0173) (3.1864, 13.9938) (3.1663, 13.9703) (3.1463, 13.9468) (3.1265, 13.9232) (3.1068, 13.8995) (3.0872, 13.8758) (3.0678, 13.852) (3.0485, 13.8281) (3.0294, 13.8042) (3.0104, 13.7803) (2.9915, 13.7562) (2.9728, 13.7321) (2.9543, 13.708) (2.9359, 13.6838) (2.9176, 13.6595) (2.8996, 13.6352) (2.8816, 13.6108) (2.8638, 13.5864) (2.8462, 13.5619) (2.8287, 13.5374) (2.8114, 13.5128) (2.7943, 13.4881) (2.7773, 13.4634) (2.7605, 13.4386) (2.7439, 13.4138) (2.7274, 13.3889) (2.7111, 13.3639) (2.695, 13.3389) (2.679, 13.3138) (2.6632, 13.2887) (2.6476, 13.2635) (2.6322, 13.2382) (2.617, 13.2129) (2.602, 13.1876) (2.5871, 13.1621) (2.5725, 13.1367) (2.558, 13.1111) (2.5438, 13.0855) (2.5297, 13.0599) (2.5159, 13.0341) (2.5023, 13.0083) (2.4889, 12.9825) (2.4758, 12.9566) (2.4628, 12.9306) (2.4501, 12.9046) (2.4376, 12.8785) (2.4253, 12.8523) (2.4133, 12.8261) (2.4015, 12.7998) (2.3901, 12.7734) (2.3791, 12.747) (2.3684, 12.7204) (2.3581, 12.6937) (2.348, 12.667) (2.3381, 12.6403) (2.3284, 12.6135) (2.3189, 12.5867) (2.31, 12.5598) (2.3018, 12.5327) (2.2961, 12.5108) (2.2924, 12.4943) (2.2902, 12.4832) (2.2892, 12.4776) knots -1 -1 -1 -1 -1 -1 -0.98571429 -0.97142857 -0.95714286 -0.94285714 -0.92857143 -0.91428571 -0.9 -0.88571429 -0.87142857 -0.85714286 -0.84285714 -0.82857143 -0.81428571 -0.8 -0.78571429 -0.77142857 -0.75714286 -0.74285714 -0.72857143 -0.71428571 -0.7 -0.68571429 -0.67142857 -0.65714286 -0.64285714 -0.62857143 -0.61428571 -0.6 -0.58571429 -0.57142857 -0.55714286 -0.54285714 -0.52857143 -0.51428571 -0.5 -0.48571429 -0.47142857 -0.45714286 -0.44285714 -0.42857143 -0.41428571 -0.4 -0.38571429 -0.37142857 -0.35714286 -0.34285714 -0.32857143 -0.31428571 -0.3 -0.28571429 -0.27142857 -0.25714286 -0.24285714 -0.22857143 -0.21428571 -0.2 -0.18571429 -0.17142857 -0.15714286 -0.14285714 -0.12857143 -0.11428571 -0.1 -0.08571429 -0.07142857 -0.05714286 -0.04285714 -0.02857143 -0.01428571 0 0 0 0 0 0
  line L11 (2.2892, 12.4776) -> (2.2006, 11.9985)
  arc A23 (2.0851, 11.9182) -> (2.2006, 11.9985) centre (2.1023, 12.0167) ccw
  arc A24 (2.0851, 11.9182) -> (1.0706, 12.0517) centre (0, 0) ccw
  arc A25 (0.9798, 12.1592) -> (1.0706, 12.0517) centre (1.0795, 12.1513) ccw
  line L12 (0.9798, 12.1592) -> (1.0183, 12.6449)
  spline S12 degree 5 poles (1.0183, 12.6449) (1.0187, 12.6506) (1.0195, 12.6618) (1.0202, 12.6788) (1.0203, 12.7014) (1.0195, 12.7297) (1.0178, 12.758) (1.0156, 12.7864) (1.0131, 12.8147) (1.0105, 12.8431) (1.0076, 12.8715) (1.0045, 12.8999) (1.0011, 12.9284) (0.9973, 12.9568) (0.9932, 12.9852) (0.9886, 13.0137) (0.9838, 13.0421) (0.9787, 13.0705) (0.9733, 13.099) (0.9678, 13.1274) (0.962, 13.1559) (0.956, 13.1843) (0.9498, 13.2127) (0.9433, 13.2412) (0.9366, 13.2696) (0.9297, 13.298) (0.9226, 13.3264) (0.9152, 13.3549) (0.9076, 13.3833) (0.8999, 13.4117) (0.8919, 13.4401) (0.8838, 13.4684) (0.8754, 13.4968) (0.8669, 13.5252) (0.8581, 13.5535) (0.8492, 13.5819) (0.8401, 13.6102) (0.8308, 13.6385) (0.8214, 13.6669) (0.8117, 13.6952) (0.8019, 13.7234) (0.7919, 13.7517) (0.7817, 13.78) (0.7714, 13.8082) (0.7609, 13.8365) (0.7502, 13.8647) (0.7393, 13.8929) (0.7283, 13.9211) (0.7171, 13.9492) (0.7058, 13.9774) (0.6943, 14.0055) (0.6826, 14.0337) (0.6708, 14.0618) (0.6588, 14.0898) (0.6467, 14.1179) (0.6344, 14.146) (0.6219, 14.174) (0.6093, 14.202) (0.5966, 14.23) (0.5837, 14.2579) (0.5706, 14.2859) (0.5574, 14.3138) (0.544, 14.3417) (0.5305, 14.3696) (0.5169, 14.3975) (0.5031, 14.4253) (0.4891, 14.4531) (0.4751, 14.4809) (0.4608, 14.5087) (0.4465, 14.5364) (0.4319, 14.5641) (0.4202, 14.5863) (0.4114, 14.6029) (0.4054, 14.6139) (0.4024, 14.6195) knots 0 0 0 0 0 0 0.01428571 0.02857143 0.04285714 0.05714286 0.07142857 0.08571429 0.1 0.11428571 0.12857143 0.14285714 0.15714286 0.17142857 0.18571429 0.2 0.21428571 0.22857143 0.24285714 0.25714286 0.27142857 0.28571429 0.3 0.31428571 0.32857143 0.34285714 0.35714286 0.37142857 0.38571429 0.4 0.41428571 0.42857143 0.44285714 0.45714286 0.47142857 0.48571429 0.5 0.51428571 0.52857143 0.54285714 0.55714286 0.57142857 0.58571429 0.6 0.61428571 0.62857143 0.64285714 0.65714286 0.67142857 0.68571429 0.7 0.71428571 0.72857143 0.74285714 0.75714286 0.77142857 0.78571429 0.8 0.81428571 0.82857143 0.84285714 0.85714286 0.87142857 0.88571429 0.9 0.91428571 0.92857143 0.94285714 0.95714286 0.97142857 0.98571429 1 1 1 1 1 1
  arc A26 (0.4024, 14.6195) -> (-0.4024, 14.6195) centre (0, 0) ccw
  spline S13 degree 5 poles (-0.4024, 14.6195) (-0.4054, 14.6139) (-0.4114, 14.6029) (-0.4202, 14.5863) (-0.4319, 14.5641) (-0.4465, 14.5364) (-0.4608, 14.5087) (-0.4751, 14.4809) (-0.4891, 14.4531) (-0.5031, 14.4253) (-0.5169, 14.3975) (-0.5305, 14.3696) (-0.544, 14.3417) (-0.5574, 14.3138) (-0.5706, 14.2859) (-0.5837, 14.2579) (-0.5966, 14.23) (-0.6093, 14.202) (-0.6219, 14.174) (-0.6344, 14.146) (-0.6467, 14.1179) (-0.6588, 14.0898) (-0.6708, 14.0618) (-0.6826, 14.0337) (-0.6943, 14.0055) (-0.7058, 13.9774) (-0.7171, 13.9492) (-0.7283, 13.9211) (-0.7393, 13.8929) (-0.7502, 13.8647) (-0.7609, 13.8365) (-0.7714, 13.8082) (-0.7817, 13.78) (-0.7919, 13.7517) (-0.8019, 13.7234) (-0.8117, 13.6952) (-0.8214, 13.6669) (-0.8308, 13.6385) (-0.8401, 13.6102) (-0.8492, 13.5819) (-0.8581, 13.5535) (-0.8669, 13.5252) (-0.8754, 13.4968) (-0.8838, 13.4684) (-0.8919, 13.4401) (-0.8999, 13.4117) (-0.9076, 13.3833) (-0.9152, 13.3549) (-0.9226, 13.3264) (-0.9297, 13.298) (-0.9366, 13.2696) (-0.9433, 13.2412) (-0.9498, 13.2127) (-0.956, 13.1843) (-0.962, 13.1559) (-0.9678, 13.1274) (-0.9733, 13.099) (-0.9787, 13.0705) (-0.9838, 13.0421) (-0.9886, 13.0137) (-0.9932, 12.9852) (-0.9973, 12.9568) (-1.0011, 12.9284) (-1.0045, 12.8999) (-1.0076, 12.8715) (-1.0105, 12.8431) (-1.0131, 12.8147) (-1.0156, 12.7864) (-1.0178, 12.758) (-1.0195, 12.7297) (-1.0203, 12.7014) (-1.0202, 12.6788) (-1.0195, 12.6618) (-1.0187, 12.6506) (-1.0183, 12.6449) knots -1 -1 -1 -1 -1 -1 -0.98571429 -0.97142857 -0.95714286 -0.94285714 -0.92857143 -0.91428571 -0.9 -0.88571429 -0.87142857 -0.85714286 -0.84285714 -0.82857143 -0.81428571 -0.8 -0.78571429 -0.77142857 -0.75714286 -0.74285714 -0.72857143 -0.71428571 -0.7 -0.68571429 -0.67142857 -0.65714286 -0.64285714 -0.62857143 -0.61428571 -0.6 -0.58571429 -0.57142857 -0.55714286 -0.54285714 -0.52857143 -0.51428571 -0.5 -0.48571429 -0.47142857 -0.45714286 -0.44285714 -0.42857143 -0.41428571 -0.4 -0.38571429 -0.37142857 -0.35714286 -0.34285714 -0.32857143 -0.31428571 -0.3 -0.28571429 -0.27142857 -0.25714286 -0.24285714 -0.22857143 -0.21428571 -0.2 -0.18571429 -0.17142857 -0.15714286 -0.14285714 -0.12857143 -0.11428571 -0.1 -0.08571429 -0.07142857 -0.05714286 -0.04285714 -0.02857143 -0.01428571 0 0 0 0 0 0
  line L13 (-1.0183, 12.6449) -> (-0.9798, 12.1592)
  arc A27 (-1.0706, 12.0517) -> (-0.9798, 12.1592) centre (-1.0795, 12.1513) ccw
  arc A28 (-1.0706, 12.0517) -> (-2.0851, 11.9182) centre (0, 0) ccw
  arc A29 (-2.2006, 11.9985) -> (-2.0851, 11.9182) centre (-2.1023, 12.0167) ccw
  line L14 (-2.2006, 11.9985) -> (-2.2892, 12.4776)
  spline S14 degree 5 poles (-2.2892, 12.4776) (-2.2902, 12.4832) (-2.2924, 12.4943) (-2.2961, 12.5108) (-2.3018, 12.5327) (-2.31, 12.5598) (-2.3189, 12.5867) (-2.3284, 12.6135) (-2.3381, 12.6403) (-2.348, 12.667) (-2.3581, 12.6937) (-2.3684, 12.7204) (-2.3791, 12.747) (-2.3901, 12.7734) (-2.4015, 12.7998) (-2.4133, 12.8261) (-2.4253, 12.8523) (-2.4376, 12.8785) (-2.4501, 12.9046) (-2.4628, 12.9306) (-2.4758, 12.9566) (-2.4889, 12.9825) (-2.5023, 13.0083) (-2.5159, 13.0341) (-2.5297, 13.0599) (-2.5438, 13.0855) (-2.558, 13.1111) (-2.5725, 13.1367) (-2.5871, 13.1621) (-2.602, 13.1876) (-2.617, 13.2129) (-2.6322, 13.2382) (-2.6476, 13.2635) (-2.6632, 13.2887) (-2.679, 13.3138) (-2.695, 13.3389) (-2.7111, 13.3639) (-2.7274, 13.3889) (-2.7439, 13.4138) (-2.7605, 13.4386) (-2.7773, 13.4634) (-2.7943, 13.4881) (-2.8114, 13.5128) (-2.8287, 13.5374) (-2.8462, 13.5619) (-2.8638, 13.5864) (-2.8816, 13.6108) (-2.8996, 13.6352) (-2.9176, 13.6595) (-2.9359, 13.6838) (-2.9543, 13.708) (-2.9728, 13.7321) (-2.9915, 13.7562) (-3.0104, 13.7803) (-3.0294, 13.8042) (-3.0485, 13.8281) (-3.0678, 13.852) (-3.0872, 13.8758) (-3.1068, 13.8995) (-3.1265, 13.9232) (-3.1463, 13.9468) (-3.1663, 13.9703) (-3.1864, 13.9938) (-3.2067, 14.0173) (-3.2271, 14.0406) (-3.2476, 14.064) (-3.2683, 14.0872) (-3.2891, 14.1104) (-3.31, 14.1336) (-3.3311, 14.1566) (-3.3522, 14.1796) (-3.3693, 14.198) (-3.3822, 14.2118) (-3.3908, 14.2209) (-3.3951, 14.2255) knots 0 0 0 0 0 0 0.01428571 0.02857143 0.04285714 0.05714286 0.07142857 0.08571429 0.1 0.11428571 0.12857143 0.14285714 0.15714286 0.17142857 0.18571429 0.2 0.21428571 0.22857143 0.24285714 0.25714286 0.27142857 0.28571429 0.3 0.31428571 0.32857143 0.34285714 0.35714286 0.37142857 0.38571429 0.4 0.41428571 0.42857143 0.44285714 0.45714286 0.47142857 0.48571429 0.5 0.51428571 0.52857143 0.54285714 0.55714286 0.57142857 0.58571429 0.6 0.61428571 0.62857143 0.64285714 0.65714286 0.67142857 0.68571429 0.7 0.71428571 0.72857143 0.74285714 0.75714286 0.77142857 0.78571429 0.8 0.81428571 0.82857143 0.84285714 0.85714286 0.87142857 0.88571429 0.9 0.91428571 0.92857143 0.94285714 0.95714286 0.97142857 0.98571429 1 1 1 1 1 1
  arc A30 (-3.3951, 14.2255) -> (-4.1725, 14.0172) centre (0, 0) ccw
  spline S15 degree 5 poles (-4.1725, 14.0172) (-4.174, 14.011) (-4.1768, 13.9988) (-4.1811, 13.9805) (-4.1867, 13.9561) (-4.1935, 13.9255) (-4.2002, 13.895) (-4.2068, 13.8645) (-4.2132, 13.834) (-4.2195, 13.8036) (-4.2256, 13.7731) (-4.2316, 13.7427) (-4.2374, 13.7122) (-4.2431, 13.6818) (-4.2486, 13.6514) (-4.254, 13.6211) (-4.2592, 13.5907) (-4.2643, 13.5604) (-4.2692, 13.53) (-4.274, 13.4998) (-4.2786, 13.4695) (-4.2831, 13.4392) (-4.2874, 13.409) (-4.2915, 13.3788) (-4.2955, 13.3486) (-4.2993, 13.3185) (-4.303, 13.2883) (-4.3065, 13.2582) (-4.3099, 13.2281) (-4.3131, 13.1981) (-4.3161, 13.1681) (-4.3189, 13.1381) (-4.3216, 13.1081) (-4.3241, 13.0782) (-4.3264, 13.0483) (-4.3286, 13.0184) (-4.3306, 12.9886) (-4.3324, 12.9588) (-4.3341, 12.929) (-4.3355, 12.8993) (-4.3368, 12.8696) (-4.3379, 12.84) (-4.3388, 12.8103) (-4.3395, 12.7808) (-4.3401, 12.7512) (-4.3404, 12.7218) (-4.3405, 12.6923) (-4.3405, 12.6629) (-4.3403, 12.6336) (-4.3398, 12.6043) (-4.3391, 12.575) (-4.3383, 12.5458) (-4.3371, 12.5167) (-4.3358, 12.4876) (-4.3342, 12.4586) (-4.3324, 12.4296) (-4.3304, 12.4007) (-4.3282, 12.3719) (-4.3258, 12.3431) (-4.3231, 12.3144) (-4.3201, 12.2857) (-4.3168, 12.2572) (-4.3131, 12.2287) (-4.3091, 12.2004) (-4.3047, 12.1722) (-4.3001, 12.144) (-4.2953, 12.1159) (-4.2903, 12.0878) (-4.2851, 12.0599) (-4.2794, 12.0321) (-4.2729, 12.0045) (-4.2669, 11.9827) (-4.2619, 11.9665) (-4.2582, 11.9558) (-4.2563, 11.9505) knots -1 -1 -1 -1 -1 -1 -0.98571429 -0.97142857 -0.95714286 -0.94285714 -0.92857143 -0.91428571 -0.9 -0.88571429 -0.87142857 -0.85714286 -0.84285714 -0.82857143 -0.81428571 -0.8 -0.78571429 -0.77142857 -0.75714286 -0.74285714 -0.72857143 -0.71428571 -0.7 -0.68571429 -0.67142857 -0.65714286 -0.64285714 -0.62857143 -0.61428571 -0.6 -0.58571429 -0.57142857 -0.55714286 -0.54285714 -0.52857143 -0.51428571 -0.5 -0.48571429 -0.47142857 -0.45714286 -0.44285714 -0.42857143 -0.41428571 -0.4 -0.38571429 -0.37142857 -0.35714286 -0.34285714 -0.32857143 -0.31428571 -0.3 -0.28571429 -0.27142857 -0.25714286 -0.24285714 -0.22857143 -0.21428571 -0.2 -0.18571429 -0.17142857 -0.15714286 -0.14285714 -0.12857143 -0.11428571 -0.1 -0.08571429 -0.07142857 -0.05714286 -0.04285714 -0.02857143 -0.01428571 0 0 0 0 0 0
  line L15 (-4.2563, 11.9505) -> (-4.0935, 11.4913)
  arc A31 (-4.1534, 11.364) -> (-4.0935, 11.4913) centre (-4.1877, 11.4579) ccw
  arc A32 (-4.1534, 11.364) -> (-5.0987, 10.9724) centre (0, 0) ccw
  arc A33 (-5.2311, 11.0201) -> (-5.0987, 10.9724) centre (-5.1408, 11.0631) ccw
  line L16 (-5.2311, 11.0201) -> (-5.4406, 11.46)
  spline S16 degree 5 poles (-5.4406, 11.46) (-5.443, 11.4651) (-5.448, 11.4752) (-5.4559, 11.4902) (-5.4671, 11.5099) (-5.482, 11.534) (-5.4976, 11.5577) (-5.5137, 11.5811) (-5.53, 11.6045) (-5.5465, 11.6277) (-5.5631, 11.6509) (-5.58, 11.674) (-5.5972, 11.6969) (-5.6147, 11.7196) (-5.6325, 11.7421) (-5.6507, 11.7645) (-5.6691, 11.7867) (-5.6877, 11.8087) (-5.7066, 11.8307) (-5.7256, 11.8526) (-5.7448, 11.8743) (-5.7642, 11.8959) (-5.7838, 11.9175) (-5.8036, 11.9389) (-5.8236, 11.9601) (-5.8439, 11.9813) (-5.8643, 12.0023) (-5.8848, 12.0232) (-5.9056, 12.0441) (-5.9265, 12.0648) (-5.9476, 12.0854) (-5.9689, 12.1059) (-5.9903, 12.1263) (-6.0119, 12.1466) (-6.0336, 12.1668) (-6.0555, 12.1869) (-6.0775, 12.2069) (-6.0998, 12.2267) (-6.1221, 12.2465) (-6.1446, 12.2662) (-6.1673, 12.2858) (-6.1901, 12.3053) (-6.213, 12.3247) (-6.2361, 12.344) (-6.2593, 12.3632) (-6.2827, 12.3822) (-6.3062, 12.4012) (-6.3298, 12.4202) (-6.3536, 12.439) (-6.3775, 12.4577) (-6.4015, 12.4763) (-6.4257, 12.4948) (-6.45, 12.5132) (-6.4744, 12.5316) (-6.4989, 12.5498) (-6.5236, 12.5679) (-6.5484, 12.586) (-6.5733, 12.6039) (-6.5983, 12.6218) (-6.6235, 12.6396) (-6.6488, 12.6572) (-6.6742, 12.6748) (-6.6997, 12.6923) (-6.7253, 12.7097) (-6.7511, 12.727) (-6.777, 12.7442) (-6.8029, 12.7613) (-6.829, 12.7783) (-6.8552, 12.7953) (-6.8816, 12.8121) (-6.908, 12.8289) (-6.9292, 12.8422) (-6.9452, 12.8521) (-6.9559, 12.8587) (-6.9612, 12.862) knots 0 0 0 0 0 0 0.01428571 0.02857143 0.04285714 0.05714286 0.07142857 0.08571429 0.1 0.11428571 0.12857143 0.14285714 0.15714286 0.17142857 0.18571429 0.2 0.21428571 0.22857143 0.24285714 0.25714286 0.27142857 0.28571429 0.3 0.31428571 0.32857143 0.34285714 0.35714286 0.37142857 0.38571429 0.4 0.41428571 0.42857143 0.44285714 0.45714286 0.47142857 0.48571429 0.5 0.51428571 0.52857143 0.54285714 0.55714286 0.57142857 0.58571429 0.6 0.61428571 0.62857143 0.64285714 0.65714286 0.67142857 0.68571429 0.7 0.71428571 0.72857143 0.74285714 0.75714286 0.77142857 0.78571429 0.8 0.81428571 0.82857143 0.84285714 0.85714286 0.87142857 0.88571429 0.9 0.91428571 0.92857143 0.94285714 0.95714286 0.97142857 0.98571429 1 1 1 1 1 1
  arc A34 (-6.9612, 12.862) -> (-7.6583, 12.4596) centre (0, 0) ccw
  spline S17 degree 5 poles (-7.6583, 12.4596) (-7.6581, 12.4533) (-7.6577, 12.4408) (-7.657, 12.422) (-7.6561, 12.3969) (-7.6548, 12.3657) (-7.6534, 12.3344) (-7.6519, 12.3033) (-7.6502, 12.2722) (-7.6483, 12.2411) (-7.6464, 12.2101) (-7.6442, 12.1792) (-7.642, 12.1483) (-7.6396, 12.1174) (-7.6371, 12.0866) (-7.6344, 12.0559) (-7.6316, 12.0252) (-7.6287, 11.9946) (-7.6256, 11.9641) (-7.6224, 11.9336) (-7.619, 11.9031) (-7.6155, 11.8728) (-7.6118, 11.8424) (-7.608, 11.8122) (-7.604, 11.782) (-7.5999, 11.7519) (-7.5957, 11.7218) (-7.5913, 11.6918) (-7.5867, 11.6619) (-7.582, 11.6321) (-7.5771, 11.6023) (-7.5721, 11.5726) (-7.567, 11.543) (-7.5617, 11.5134) (-7.5562, 11.4839) (-7.5505, 11.4545) (-7.5447, 11.4252) (-7.5388, 11.3959) (-7.5327, 11.3667) (-7.5264, 11.3376) (-7.5199, 11.3086) (-7.5133, 11.2797) (-7.5065, 11.2509) (-7.4996, 11.2221) (-7.4924, 11.1935) (-7.4851, 11.1649) (-7.4777, 11.1364) (-7.47, 11.108) (-7.4622, 11.0798) (-7.4542, 11.0516) (-7.4459, 11.0235) (-7.4375, 10.9955) (-7.4289, 10.9677) (-7.4201, 10.9399) (-7.411, 10.9123) (-7.4018, 10.8848) (-7.3924, 10.8574) (-7.3828, 10.8301) (-7.373, 10.8029) (-7.363, 10.7759) (-7.3527, 10.749) (-7.3421, 10.7222) (-7.3312, 10.6957) (-7.3199, 10.6694) (-7.3084, 10.6433) (-7.2967, 10.6172) (-7.2848, 10.5913) (-7.2727, 10.5655) (-7.2604, 10.5399) (-7.2477, 10.5145) (-7.2343, 10.4896) (-7.2229, 10.4701) (-7.2138, 10.4557) (-7.2075, 10.4463) (-7.2043, 10.4417) knots -1 -1 -1 -1 -1 -1 -0.98571429 -0.97142857 -0.95714286 -0.94285714 -0.92857143 -0.91428571 -0.9 -0.88571429 -0.87142857 -0.85714286 -0.84285714 -0.82857143 -0.81428571 -0.8 -0.78571429 -0.77142857 -0.75714286 -0.74285714 -0.72857143 -0.71428571 -0.7 -0.68571429 -0.67142857 -0.65714286 -0.64285714 -0.62857143 -0.61428571 -0.6 -0.58571429 -0.57142857 -0.55714286 -0.54285714 -0.52857143 -0.51428571 -0.5 -0.48571429 -0.47142857 -0.45714286 -0.44285714 -0.42857143 -0.41428571 -0.4 -0.38571429 -0.37142857 -0.35714286 -0.34285714 -0.32857143 -0.31428571 -0.3 -0.28571429 -0.27142857 -0.25714286 -0.24285714 -0.22857143 -0.21428571 -0.2 -0.18571429 -0.17142857 -0.15714286 -0.14285714 -0.12857143 -0.11428571 -0.1 -0.08571429 -0.07142857 -0.05714286 -0.04285714 -0.02857143 -0.01428571 0 0 0 0 0 0
  line L17 (-7.2043, 10.4417) -> (-6.9282, 10.0403)
  arc A35 (-6.9531, 9.9018) -> (-6.9282, 10.0403) centre (-7.0105, 9.9836) ccw
  arc A36 (-6.9531, 9.9018) -> (-7.7648, 9.2789) centre (0, 0) ccw
  arc A37 (-7.905, 9.2907) -> (-7.7648, 9.2789) centre (-7.829, 9.3556) ccw
  line L18 (-7.905, 9.2907) -> (-8.2213, 9.6613)